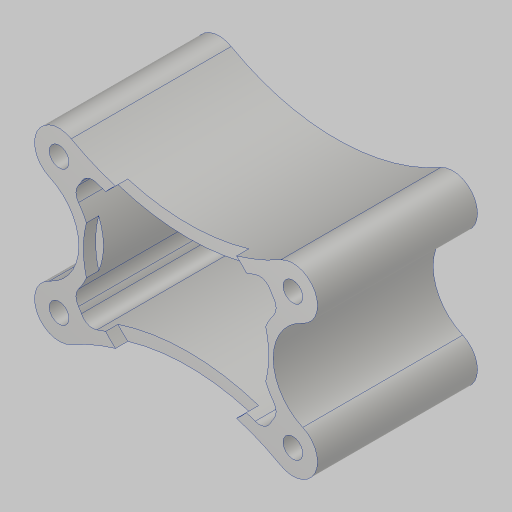
# Autodesk Inventor part: AR-009
Saved by Autodesk Inventor 2023.5 (Build 275446000, 446)
## iProperties
Created: 2025-01-23
Part Number: AR-009
Material: Aluminum 6061
Document SubType Name: Modeling
Designer: mavericks
Density: 2.7 g/cm^3
Appearance: Aluminum - Flat
Mass: 87.8054 g
Surface Area: 188.019 cm^2
Volume: 32.5205 cm^3
Author: mavericks
Autodesk Inventor part; units mm, degrees
ref_plane "YZ Plane" through (0, 0, 0) normal (1, 0, 0) x (0, 1, 0)
ref_plane "XZ Plane" through (0, 0, 0) normal (0, 1, 0) x (-1, 0, 0)
ref_plane "XY Plane" through (0, 0, 0) normal (0, 0, 1) x (1, 0, 0)
sketch "Sketch1" plane through (0, 0, 0) normal (0, 0, 1) x (1, 0, 0)
  line L0 (-30.1625, -17.4625) -> (30.1625, -17.4625) construction
  line L1 (30.1625, -17.4625) -> (30.1625, 17.4625) construction
  line L2 (30.1625, 17.4625) -> (-30.1625, 17.4625) construction
  line L3 (-30.1625, 17.4625) -> (-30.1625, -17.4625) construction
  line L4 (-30.1625, -17.4625) -> (30.1625, 17.4625) construction
  line L5 (30.1625, -17.4625) -> (-30.1625, 17.4625) construction
  circle A0 centre (-30.1625, -17.4625) radius 6.35 construction
  circle A1 centre (-30.1625, 17.4625) radius 6.35 construction
  circle A2 centre (30.1625, 17.4625) radius 6.35 construction
  circle A3 centre (30.1625, -17.4625) radius 6.35 construction
  circle A4 centre (0, 0) radius 15.875 construction
  arc A5 (27.0369, -22.99) -> (-27.0369, -22.99) centre (0, -70.8025) ccw
  arc A6 (32.7003, 11.6417) -> (32.7003, -11.6417) centre (37.7759, 0) ccw
  arc A7 (-27.0369, 22.99) -> (27.0369, 22.99) centre (0, 70.8025) ccw
  arc A8 (-32.7003, -11.6417) -> (-32.7003, 11.6417) centre (-37.7759, 0) ccw
  arc A9 (-31.4314, -14.5521) -> (-31.4314, 14.5521) centre (-37.7759, 0) ccw
  arc A10 (37.6958, -26.5879) -> (-37.6958, -26.5879) centre (0, -70.8025) ccw
  arc A11 (31.4314, 14.5521) -> (31.4314, -14.5521) centre (37.7759, 0) ccw
  arc A12 (-37.6958, 26.5879) -> (37.6958, 26.5879) centre (0, 70.8025) ccw
  arc A13 (-27.0369, 22.99) -> (-32.7003, 11.6417) centre (-30.1625, 17.4625) ccw
  arc A14 (-27.2047, 11.8434) -> (-23.8219, 17.808) centre (-30.1625, 17.4625) ccw
  arc A15 (32.7003, 11.6417) -> (27.0369, 22.99) centre (30.1625, 17.4625) ccw
  arc A16 (23.8219, 17.808) -> (27.2047, 11.8434) centre (30.1625, 17.4625) ccw
  arc A17 (27.0369, -22.99) -> (32.7003, -11.6417) centre (30.1625, -17.4625) ccw
  arc A18 (27.2047, -11.8434) -> (23.8219, -17.808) centre (30.1625, -17.4625) ccw
  arc A19 (-32.7003, -11.6417) -> (-27.0369, -22.99) centre (-30.1625, -17.4625) ccw
  arc A20 (-23.8219, -17.808) -> (-27.2047, -11.8434) centre (-30.1625, -17.4625) ccw
  dimension "d0" = 60.325
  dimension "d1" = 34.925
  dimension "d2" = 12.7
  dimension "d3" = 12.7
  dimension "d4" = 12.7
  dimension "d5" = 12.7
  dimension "d6" = 31.75
  dimension "d7" = 12.7
  dimension "d8" = 12.7
  dimension "d9" = 3.175
  dimension "d10" = 3.175
  constraints: 56 point on circle, 21 centre point, 17 coincident, 12 end point, 10 tangent, 2 equal radius, 2 midpoint, 2 parallel, 1 horizontal, 1 perpendicular
  measures "d0" distance of L2.end L1.end
  measures "d1" distance of L1.end L0.end
  measures "d2" diameter of A0
  measures "d3" diameter of A1
  measures "d4" diameter of A2
  measures "d5" diameter of A3
  measures "d6" diameter of A4
  measures "d7" radius of A8
  measures "d8" radius of A6
  measures "d9" radial gap between concentric circles of A8 A9
  measures "d10" radial gap between concentric circles of A7 A12
extrude "Extrusion1" add sketch "Sketch1" along normal blind 41.275 contours A5 A19 A10 A17 | A10 A18 A11 A16 A12 A15 A6 A17 | A19 A8 A13 A12 A14 A9 A20 A10 | A12 A13 A7 A15
fillet "Fillet1" radius 3.175 8 edges at (-27.2047, -11.8434, 20.6375) (-27.2047, 11.8434, 20.6375) (-23.8219, 17.808, 20.6375) (23.8219, 17.808, 20.6375) (27.2047, 11.8434, 20.6375) (27.2047, -11.8434, 20.6375) (23.8219, -17.808, 20.6375) (-23.8219, -17.808, 20.6375)
hole "Hole1" at (30.1625, 17.4625, 0) at (30.1625, -17.4625, 0) at (-30.1625, -17.4625, 0) at (-30.1625, 17.4625, 0) direction (0, 0, 1) diameter 5.1054 end through all clearance for "Flat Head Machine Screw (82)" size "#10" standard "Ansi Unified Screw Threads"
sketch "Sketch3" plane through (0, 0, 41.275) normal (0, 0, 1) x (1, 0, 0)
  circle A0 centre (0, 0) radius 23.9395
  dimension "d21" = 47.879
  constraints: 1 centre point, 1 coincident
  measures "d21" diameter of A0
extrude "Extrusion2" cut sketch "Sketch3" against normal blind 3.175
equation "\"d8\" = d7"
equation "\"d10\" = d9"
body "Solid1"
